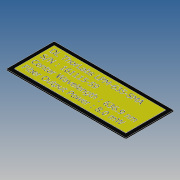
# Autodesk Inventor part: P131
Saved by Autodesk Inventor 2019 (Build 230136000, 136)
## iProperties
Created: 2017-01-31
Part Number: P131
Material: Generic
Document SubType Name: Modeling
Designer: serge.amoos
Density: 1 g/cm^3
Appearance: Smooth - Black
Description: Plaquette Thorlabs
Author: serge.amoos
Autodesk Inventor part; units mm, degrees
(part 1 of 3)
ref_plane "YZ Plane" through (0, 0, 0) normal (1, 0, 0) x (0, 1, 0)
ref_plane "XZ Plane" through (0, 0, 0) normal (0, 1, 0) x (-1, 0, 0)
ref_plane "XY Plane" through (0, 0, 0) normal (0, 0, 1) x (1, 0, 0)
sketch "Sketch1" plane through (0, 0, 0) normal (0, 0, 1) x (1, 0, 0)
  line L0 (-24.1301, 0) -> (24.0032, 0)
  line L1 (0, -8.4) -> (0, 8.4)
  line L2 (-15, 6) -> (15, 6)
  line L3 (15, 6) -> (15, -6)
  line L4 (15, -6) -> (-15, -6)
  line L5 (-15, -6) -> (-15, 6)
  point P0 (0, 0)
  point P1 (0, 6)
  point P2 (15, 0)
  dimension "d0" = 30
  dimension "d1" = 12
  constraints: 8 end point, 2 midpoint, 2 parallel, 2 point on line, 1 horizontal, 1 perpendicular
  measures "d0" distance of L2.start L2.end
  measures "d1" distance of L2.end L3.end
extrude "Extrusion1" add sketch "Sketch1" along normal blind 0.4
sketch "Sketch2" plane through (0, 0, 0.4) normal (0, 0, 1) x (1, 0, 0)
  line L0 (14, 5) -> (14, -5)
  line L1 (14, -5) -> (-14, -5)
  line L2 (-14, -5) -> (-14, 5)
  line L3 (-14, 5) -> (14, 5)
  line L4 (15, -6) -> (-15, -6)
  line L5 (-15, -6) -> (-15, 6)
  line L6 (-15, 6) -> (15, 6)
  line L7 (15, 6) -> (15, -6)
  point P0 (0, 0)
  dimension "d10" = 1
  dimension "d11" = 1
  dimension "d12" = 1
  dimension "d13" = 1
  constraints: 8 end point
  measures "d10" distance between parallel lines of L3 L6
  measures "d11" distance between parallel lines of L7 L0
  measures "d12" distance between parallel lines of L4 L1
  measures "d13" distance between parallel lines of L5 L2
extrude "Extrusion4" cut sketch "Sketch2" against normal blind 0.1
sketch "Sketch3" plane through (0, 0, 0.4) normal (0, 0, 1) x (1, 0, 0)
  line L0 (-13.4008, 7.7124) -> (17.127, 7.7124) construction
  line L1 (17.127, 7.7124) -> (17.127, -7.7124) construction
  line L2 (17.127, -7.7124) -> (-13.4008, -7.7124) construction
  line L3 (-13.4008, -7.7124) -> (-13.4008, 7.7124) construction
  line L4 (-23.9778, 0) -> (23.9778, 0)
  line L5 (0, -8.4) -> (0, 8.4)
  line L6 (14, -5) -> (-14, -5)
  line L7 (-14, -5) -> (-14, 5)
  line L8 (-14, 5) -> (14, 5)
  line L9 (14, 5) -> (14, -5)
  spline S0 degree 2 poles (-12.1551, 3.6187) (-12.1551, 3.427) (-12.3105, 3.1184) (-12.441, 3.0321) knots 0 0 0 1 2 2 2
  spline S1 degree 2 poles (-12.441, 3.0321) (-12.5477, 2.9652) (-12.7666, 2.9198) (-12.9368, 2.9198) knots 0 0 0 1 2 2 2
  line L10 (-12.9368, 2.9198) -> (-13.259, 2.9198)
  line L11 (-13.259, 2.9198) -> (-13.259, 4.3198)
  line L12 (-13.259, 4.3198) -> (-12.9402, 4.3198)
  spline S2 degree 2 poles (-12.9402, 4.3198) (-12.7428, 4.3198) (-12.5182, 4.2608) (-12.4387, 4.2086) knots 0 0 0 1 2 2 2
  spline S3 degree 2 poles (-12.4387, 4.2086) (-12.3037, 4.119) (-12.1551, 3.8229) (-12.1551, 3.6187) knots 0 0 0 1 2 2 2
  spline S4 degree 2 poles (-12.3491, 3.621) (-12.3491, 3.7821) (-12.4558, 4.0101) (-12.5613, 4.0748) knots 0 0 0 1 2 2 2
  spline S5 degree 2 poles (-12.5613, 4.0748) (-12.6362, 4.119) (-12.8052, 4.1587) (-12.9311, 4.1587) knots 0 0 0 1 2 2 2
  line L13 (-12.9311, 4.1587) -> (-13.0729, 4.1587)
  line L14 (-13.0729, 4.1587) -> (-13.0729, 3.0809)
  line L15 (-13.0729, 3.0809) -> (-12.9311, 3.0809)
  spline S6 degree 2 poles (-12.9311, 3.0809) (-12.8075, 3.0809) (-12.6203, 3.1206) (-12.5443, 3.174) knots 0 0 0 1 2 2 2
  spline S7 degree 2 poles (-12.5443, 3.174) (-12.4467, 3.2398) (-12.3491, 3.4576) (-12.3491, 3.621) knots 0 0 0 1 2 2 2
  line L16 (-11.142, 2.9198) -> (-11.9532, 2.9198)
  line L17 (-11.9532, 2.9198) -> (-11.9532, 4.3198)
  line L18 (-11.9532, 4.3198) -> (-11.7671, 4.3198)
  line L19 (-11.7671, 4.3198) -> (-11.7671, 3.0855)
  line L20 (-11.7671, 3.0855) -> (-11.142, 3.0855)
  line L21 (-11.142, 3.0855) -> (-11.142, 2.9198)
  line L22 (-10.0676, 2.9198) -> (-10.0676, 4.1542)
  line L23 (-10.0676, 4.1542) -> (-10.5373, 4.1542)
  line L24 (-10.5373, 4.1542) -> (-10.5373, 4.3198)
  line L25 (-10.5373, 4.3198) -> (-9.4118, 4.3198)
  line L26 (-9.4118, 4.3198) -> (-9.4118, 4.1542)
  line L27 (-9.4118, 4.1542) -> (-9.8815, 4.1542)
  line L28 (-9.8815, 4.1542) -> (-9.8815, 2.9198)
  line L29 (-9.8815, 2.9198) -> (-10.0676, 2.9198)
  line L30 (-8.4588, 2.9198) -> (-8.6358, 2.9198)
  line L31 (-8.6358, 2.9198) -> (-8.6358, 3.5189)
  spline S8 degree 2 poles (-8.6358, 3.5189) (-8.6358, 3.5915) (-8.6494, 3.7163) (-8.6699, 3.7537) knots 0 0 0 1 2 2 2
  spline S9 degree 2 poles (-8.6699, 3.7537) (-8.6914, 3.7934) (-8.7686, 3.832) (-8.8344, 3.832) knots 0 0 0 1 2 2 2
  spline S10 degree 2 poles (-8.8344, 3.832) (-8.9002, 3.832) (-9.0397, 3.7616) (-9.1067, 3.7049) knots 0 0 0 1 2 2 2
  line L32 (-9.1067, 3.7049) -> (-9.1067, 2.9198)
  line L33 (-9.1067, 2.9198) -> (-9.2836, 2.9198)
  line L34 (-9.2836, 2.9198) -> (-9.2836, 4.3822)
  line L35 (-9.2836, 4.3822) -> (-9.1067, 4.3822)
  line L36 (-9.1067, 4.3822) -> (-9.1067, 3.8535)
  spline S11 degree 2 poles (-9.1067, 3.8535) (-9.0272, 3.925) (-8.8741, 3.9999) (-8.7879, 3.9999) knots 0 0 0 1 2 2 2
  spline S12 degree 2 poles (-8.7879, 3.9999) (-8.6336, 3.9999) (-8.4588, 3.7957) (-8.4588, 3.6017) knots 0 0 0 1 2 2 2
  line L37 (-8.4588, 3.6017) -> (-8.4588, 2.9198)
  spline S13 degree 2 poles (-7.347, 3.4451) (-7.347, 3.1796) (-7.6023, 2.8903) (-7.8156, 2.8903) knots 0 0 0 1 2 2 2
  spline S14 degree 2 poles (-7.8156, 2.8903) (-8.0345, 2.8903) (-8.2853, 3.1887) (-8.2853, 3.4451) knots 0 0 0 1 2 2 2
  spline S15 degree 2 poles (-8.2853, 3.4451) (-8.2853, 3.7083) (-8.0266, 3.9999) (-7.8156, 3.9999) knots 0 0 0 1 2 2 2
  spline S16 degree 2 poles (-7.8156, 3.9999) (-7.6023, 3.9999) (-7.347, 3.7095) (-7.347, 3.4451) knots 0 0 0 1 2 2 2
  spline S17 degree 2 poles (-7.5297, 3.4451) (-7.5297, 3.6493) (-7.6783, 3.8479) (-7.8156, 3.8479) knots 0 0 0 1 2 2 2
  spline S18 degree 2 poles (-7.8156, 3.8479) (-7.9529, 3.8479) (-8.1026, 3.6493) (-8.1026, 3.4451) knots 0 0 0 1 2 2 2
  spline S19 degree 2 poles (-8.1026, 3.4451) (-8.1026, 3.2466) (-7.9529, 3.0424) (-7.8156, 3.0424) knots 0 0 0 1 2 2 2
  spline S20 degree 2 poles (-7.8156, 3.0424) (-7.6794, 3.0424) (-7.5297, 3.2432) (-7.5297, 3.4451) knots 0 0 0 1 2 2 2
  line L38 (-6.6084, 3.7809) -> (-6.6175, 3.7809)
  spline S21 degree 2 poles (-6.6175, 3.7809) (-6.6379, 3.7866) (-6.6822, 3.7889) (-6.7128, 3.7889) knots 0 0 0 1 2 2 2
  spline S22 degree 2 poles (-6.7128, 3.7889) (-6.7843, 3.7889) (-6.925, 3.7265) (-6.9885, 3.6652) knots 0 0 0 1 2 2 2
  line L39 (-6.9885, 3.6652) -> (-6.9885, 2.9198)
  line L40 (-6.9885, 2.9198) -> (-7.1655, 2.9198)
  line L41 (-7.1655, 2.9198) -> (-7.1655, 3.9704)
  line L42 (-7.1655, 3.9704) -> (-6.9885, 3.9704)
  line L43 (-6.9885, 3.9704) -> (-6.9885, 3.8138)
  spline S23 degree 2 poles (-6.9885, 3.8138) (-6.8921, 3.9001) (-6.748, 3.9704) (-6.6799, 3.9704) knots 0 0 0 1 2 2 2
  spline S24 degree 2 poles (-6.6799, 3.9704) (-6.6527, 3.9704) (-6.6255, 3.9681) (-6.6084, 3.9647) knots 0 0 0 1 2 2 2
  line L44 (-6.6084, 3.9647) -> (-6.6084, 3.7809)
  line L45 (-5.6464, 2.9198) -> (-6.4576, 2.9198)
  line L46 (-6.4576, 2.9198) -> (-6.4576, 4.3198)
  line L47 (-6.4576, 4.3198) -> (-6.2715, 4.3198)
  line L48 (-6.2715, 4.3198) -> (-6.2715, 3.0855)
  line L49 (-6.2715, 3.0855) -> (-5.6464, 3.0855)
  line L50 (-5.6464, 3.0855) -> (-5.6464, 2.9198)
  spline S25 degree 2 poles (-4.9282, 3.031) (-4.9498, 3.0151) (-5.0224, 2.9584) (-5.0564, 2.9414) knots 0 0 0 1 2 2 2
  spline S26 degree 2 poles (-5.0564, 2.9414) (-5.1029, 2.9164) (-5.1903, 2.8903) (-5.2697, 2.8903) knots 0 0 0 1 2 2 2
  spline S27 degree 2 poles (-5.2697, 2.8903) (-5.3344, 2.8903) (-5.4512, 2.9391) (-5.4955, 2.9834) knots 0 0 0 1 2 2 2
  spline S28 degree 2 poles (-5.4955, 2.9834) (-5.5375, 3.0265) (-5.5885, 3.1535) (-5.5885, 3.2239) knots 0 0 0 1 2 2 2
  spline S29 degree 2 poles (-5.5885, 3.2239) (-5.5885, 3.3328) (-5.4966, 3.4871) (-5.3968, 3.5313) knots 0 0 0 1 2 2 2
  spline S30 degree 2 poles (-5.3968, 3.5313) (-5.3083, 3.5722) (-5.0678, 3.6028) (-4.9282, 3.6108) knots 0 0 0 1 2 2 2
  line L51 (-4.9282, 3.6108) -> (-4.9282, 3.6448)
  spline S31 degree 2 poles (-4.9282, 3.6448) (-4.9282, 3.7061) (-4.9657, 3.7821) (-4.9997, 3.8036) knots 0 0 0 1 2 2 2
  spline S32 degree 2 poles (-4.9997, 3.8036) (-5.0337, 3.8252) (-5.1313, 3.8388) (-5.1835, 3.8388) knots 0 0 0 1 2 2 2
  spline S33 degree 2 poles (-5.1835, 3.8388) (-5.2447, 3.8388) (-5.4104, 3.8025) (-5.4932, 3.7673) knots 0 0 0 1 2 2 2
  line L52 (-5.4932, 3.7673) -> (-5.5034, 3.7673)
  line L53 (-5.5034, 3.7673) -> (-5.5034, 3.9477)
  spline S34 degree 2 poles (-5.5034, 3.9477) (-5.4546, 3.9613) (-5.272, 3.9954) (-5.1823, 3.9954) knots 0 0 0 1 2 2 2
  spline S35 degree 2 poles (-5.1823, 3.9954) (-5.0734, 3.9954) (-4.9248, 3.9613) (-4.8658, 3.9171) knots 0 0 0 1 2 2 2
  spline S36 degree 2 poles (-4.8658, 3.9171) (-4.808, 3.874) (-4.7512, 3.7367) (-4.7512, 3.638) knots 0 0 0 1 2 2 2
  line L54 (-4.7512, 3.638) -> (-4.7512, 2.9198)
  line L55 (-4.7512, 2.9198) -> (-4.9282, 2.9198)
  line L56 (-4.9282, 2.9198) -> (-4.9282, 3.031)
  line L57 (-4.9282, 3.1785) -> (-4.9282, 3.4701)
  spline S37 degree 2 poles (-4.9282, 3.4701) (-4.9917, 3.4644) (-5.1835, 3.4451) (-5.2436, 3.427) knots 0 0 0 1 2 2 2
  spline S38 degree 2 poles (-5.2436, 3.427) (-5.314, 3.4054) (-5.4058, 3.3158) (-5.4058, 3.2364) knots 0 0 0 1 2 2 2
  spline S39 degree 2 poles (-5.4058, 3.2364) (-5.4058, 3.1456) (-5.3037, 3.0537) (-5.2062, 3.0537) knots 0 0 0 1 2 2 2
  spline S40 degree 2 poles (-5.2062, 3.0537) (-5.1234, 3.0537) (-4.9872, 3.1252) (-4.9282, 3.1785) knots 0 0 0 1 2 2 2
  spline S41 degree 2 poles (-3.6224, 3.4621) (-3.6224, 3.2046) (-3.872, 2.8903) (-4.0603, 2.8903) knots 0 0 0 1 2 2 2
  spline S42 degree 2 poles (-4.0603, 2.8903) (-4.1454, 2.8903) (-4.2668, 2.9323) (-4.3258, 2.9686) knots 0 0 0 1 2 2 2
  line L58 (-4.3258, 2.9686) -> (-4.3371, 2.9198)
  line L59 (-4.3371, 2.9198) -> (-4.5028, 2.9198)
  line L60 (-4.5028, 2.9198) -> (-4.5028, 4.3822)
  line L61 (-4.5028, 4.3822) -> (-4.3258, 4.3822)
  line L62 (-4.3258, 4.3822) -> (-4.3258, 3.8603)
  spline S43 degree 2 poles (-4.3258, 3.8603) (-4.2588, 3.9205) (-4.1034, 3.9999) (-4.0047, 3.9999) knots 0 0 0 1 2 2 2
  spline S44 degree 2 poles (-4.0047, 3.9999) (-3.8266, 3.9999) (-3.6224, 3.7151) (-3.6224, 3.4621) knots 0 0 0 1 2 2 2
  spline S45 degree 2 poles (-3.805, 3.4485) (-3.805, 3.6368) (-3.9196, 3.832) (-4.0467, 3.832) knots 0 0 0 1 2 2 2
  spline S46 degree 2 poles (-4.0467, 3.832) (-4.1182, 3.832) (-4.2657, 3.7639) (-4.3258, 3.7117) knots 0 0 0 1 2 2 2
  line L63 (-4.3258, 3.7117) -> (-4.3258, 3.1093)
  spline S47 degree 2 poles (-4.3258, 3.1093) (-4.2588, 3.0764) (-4.1556, 3.0492) (-4.0943, 3.0492) knots 0 0 0 1 2 2 2
  spline S48 degree 2 poles (-4.0943, 3.0492) (-3.9593, 3.0492) (-3.805, 3.2409) (-3.805, 3.4485) knots 0 0 0 1 2 2 2
  spline S49 degree 2 poles (-3.155, 2.8949) (-3.2605, 2.8949) (-3.4431, 2.9516) (-3.5033, 2.9834) knots 0 0 0 1 2 2 2
  line L64 (-3.5033, 2.9834) -> (-3.5033, 3.1819)
  line L65 (-3.5033, 3.1819) -> (-3.4942, 3.1819)
  spline S50 degree 2 poles (-3.4942, 3.1819) (-3.4715, 3.1638) (-3.4102, 3.1206) (-3.3592, 3.0968) knots 0 0 0 1 2 2 2
  spline S51 degree 2 poles (-3.3592, 3.0968) (-3.3149, 3.0753) (-3.206, 3.0435) (-3.1482, 3.0435) knots 0 0 0 1 2 2 2
  spline S52 degree 2 poles (-3.1482, 3.0435) (-3.1062, 3.0435) (-3.0097, 3.0628) (-2.987, 3.0787) knots 0 0 0 1 2 2 2
  spline S53 degree 2 poles (-2.987, 3.0787) (-2.9541, 3.1002) (-2.9246, 3.149) (-2.9246, 3.1989) knots 0 0 0 1 2 2 2
  spline S54 degree 2 poles (-2.9246, 3.1989) (-2.9246, 3.2613) (-2.9927, 3.326) (-3.0801, 3.3475) knots 0 0 0 1 2 2 2
  spline S55 degree 2 poles (-3.0801, 3.3475) (-3.1141, 3.3555) (-3.223, 3.3782) (-3.2695, 3.3907) knots 0 0 0 1 2 2 2
  spline S56 degree 2 poles (-3.2695, 3.3907) (-3.3898, 3.4258) (-3.4987, 3.571) (-3.4987, 3.6743) knots 0 0 0 1 2 2 2
  spline S57 degree 2 poles (-3.4987, 3.6743) (-3.4987, 3.8172) (-3.2843, 3.9954) (-3.1073, 3.9954) knots 0 0 0 1 2 2 2
  spline S58 degree 2 poles (-3.1073, 3.9954) (-3.0199, 3.9954) (-2.843, 3.9522) (-2.7828, 3.9193) knots 0 0 0 1 2 2 2
  line L66 (-2.7828, 3.9193) -> (-2.7828, 3.7299)
  line L67 (-2.7828, 3.7299) -> (-2.7919, 3.7299)
  spline S59 degree 2 poles (-2.7919, 3.7299) (-2.86, 3.7843) (-3.0256, 3.8467) (-3.1107, 3.8467) knots 0 0 0 1 2 2 2
  spline S60 degree 2 poles (-3.1107, 3.8467) (-3.1981, 3.8467) (-3.3183, 3.773) (-3.3183, 3.6992) knots 0 0 0 1 2 2 2
  spline S61 degree 2 poles (-3.3183, 3.6992) (-3.3183, 3.6323) (-3.2469, 3.5676) (-3.1674, 3.5472) knots 0 0 0 1 2 2 2
  spline S62 degree 2 poles (-3.1674, 3.5472) (-3.1289, 3.537) (-3.0313, 3.5166) (-2.978, 3.5041) knots 0 0 0 1 2 2 2
  spline S63 degree 2 poles (-2.978, 3.5041) (-2.8623, 3.4746) (-2.7443, 3.3396) (-2.7443, 3.2227) knots 0 0 0 1 2 2 2
  spline S64 degree 2 poles (-2.7443, 3.2227) (-2.7443, 3.1547) (-2.7976, 3.0344) (-2.8498, 2.9902) knots 0 0 0 1 2 2 2
  spline S65 degree 2 poles (-2.8498, 2.9902) (-2.9054, 2.9437) (-3.0472, 2.8949) (-3.155, 2.8949) knots 0 0 0 1 2 2 2
  line L68 (-1.1537, 2.9198) -> (-1.9648, 2.9198)
  line L69 (-1.9648, 2.9198) -> (-1.9648, 4.3198)
  line L70 (-1.9648, 4.3198) -> (-1.7788, 4.3198)
  line L71 (-1.7788, 4.3198) -> (-1.7788, 3.0855)
  line L72 (-1.7788, 3.0855) -> (-1.1537, 3.0855)
  line L73 (-1.1537, 3.0855) -> (-1.1537, 2.9198)
  spline S66 degree 2 poles (-0.1224, 3.8978) (-0.1224, 3.807) (-0.187, 3.6437) (-0.2449, 3.5869) knots 0 0 0 1 2 2 2
  spline S67 degree 2 poles (-0.2449, 3.5869) (-0.3175, 3.5155) (-0.5138, 3.4417) (-0.6635, 3.4417) knots 0 0 0 1 2 2 2
  line L74 (-0.6635, 3.4417) -> (-0.8212, 3.4417)
  line L75 (-0.8212, 3.4417) -> (-0.8212, 2.9198)
  line L76 (-0.8212, 2.9198) -> (-1.0073, 2.9198)
  line L77 (-1.0073, 2.9198) -> (-1.0073, 4.3198)
  line L78 (-1.0073, 4.3198) -> (-0.6556, 4.3198)
  spline S68 degree 2 poles (-0.6556, 4.3198) (-0.5308, 4.3198) (-0.3561, 4.279) (-0.2892, 4.2325) knots 0 0 0 1 2 2 2
  spline S69 degree 2 poles (-0.2892, 4.2325) (-0.2109, 4.1792) (-0.1224, 4.0146) (-0.1224, 3.8978) knots 0 0 0 1 2 2 2
  spline S70 degree 2 poles (-0.3164, 3.8921) (-0.3164, 3.9647) (-0.3663, 4.0714) (-0.4174, 4.1054) knots 0 0 0 1 2 2 2
  spline S71 degree 2 poles (-0.4174, 4.1054) (-0.4616, 4.1349) (-0.5796, 4.1587) (-0.667, 4.1587) knots 0 0 0 1 2 2 2
  line L79 (-0.667, 4.1587) -> (-0.8212, 4.1587)
  line L80 (-0.8212, 4.1587) -> (-0.8212, 3.6005)
  line L81 (-0.8212, 3.6005) -> (-0.6942, 3.6005)
  spline S72 degree 2 poles (-0.6942, 3.6005) (-0.5807, 3.6005) (-0.4412, 3.6368) (-0.3958, 3.6845) knots 0 0 0 1 2 2 2
  spline S73 degree 2 poles (-0.3958, 3.6845) (-0.3538, 3.7265) (-0.3164, 3.8252) (-0.3164, 3.8921) knots 0 0 0 1 2 2 2
  line L82 (1.2549, 2.9198) -> (1.0689, 2.9198)
  line L83 (1.0689, 2.9198) -> (1.0689, 4.1258)
  line L84 (1.0689, 4.1258) -> (0.7036, 3.3056)
  line L85 (0.7036, 3.3056) -> (0.5901, 3.3056)
  line L86 (0.5901, 3.3056) -> (0.2282, 4.1258)
  line L87 (0.2282, 4.1258) -> (0.2282, 2.9198)
  line L88 (0.2282, 2.9198) -> (0.0546, 2.9198)
  line L89 (0.0546, 2.9198) -> (0.0546, 4.3198)
  line L90 (0.0546, 4.3198) -> (0.3087, 4.3198)
  line L91 (0.3087, 4.3198) -> (0.6582, 3.5404)
  line L92 (0.6582, 3.5404) -> (0.9963, 4.3198)
  line L93 (0.9963, 4.3198) -> (1.2549, 4.3198)
  line L94 (1.2549, 4.3198) -> (1.2549, 2.9198)
  line L95 (2.0117, 3.4474) -> (1.4818, 3.4474)
  line L96 (1.4818, 3.4474) -> (1.4818, 3.6176)
  line L97 (1.4818, 3.6176) -> (2.0117, 3.6176)
  line L98 (2.0117, 3.6176) -> (2.0117, 3.4474)
  spline S74 degree 2 poles (3.0826, 3.3736) (3.0826, 3.2659) (3.0112, 3.0832) (2.951, 3.0219) knots 0 0 0 1 2 2 2
  spline S75 degree 2 poles (2.951, 3.0219) (2.8886, 2.9573) (2.7321, 2.8903) (2.6379, 2.8903) knots 0 0 0 1 2 2 2
  spline S76 degree 2 poles (2.6379, 2.8903) (2.5437, 2.8903) (2.3883, 2.9539) (2.3293, 3.0174) knots 0 0 0 1 2 2 2
  spline S77 degree 2 poles (2.3293, 3.0174) (2.2567, 3.0934) (2.175, 3.3487) (2.175, 3.5347) knots 0 0 0 1 2 2 2
  spline S78 degree 2 poles (2.175, 3.5347) (2.175, 3.7174) (2.2499, 4.0112) (2.3282, 4.1202) knots 0 0 0 1 2 2 2
  spline S79 degree 2 poles (2.3282, 4.1202) (2.4042, 4.2268) (2.6447, 4.3459) (2.8024, 4.3459) knots 0 0 0 1 2 2 2
  spline S80 degree 2 poles (2.8024, 4.3459) (2.8489, 4.3459) (2.9306, 4.3368) (2.9613, 4.3266) knots 0 0 0 1 2 2 2
  line L99 (2.9613, 4.3266) -> (2.9613, 4.1462)
  line L100 (2.9613, 4.1462) -> (2.9533, 4.1462)
  spline S81 degree 2 poles (2.9533, 4.1462) (2.9272, 4.1599) (2.8319, 4.1837) (2.7775, 4.1837) knots 0 0 0 1 2 2 2
  spline S82 degree 2 poles (2.7775, 4.1837) (2.6027, 4.1837) (2.3883, 3.9477) (2.3679, 3.7163) knots 0 0 0 1 2 2 2
  spline S83 degree 2 poles (2.3679, 3.7163) (2.4348, 3.7628) (2.5755, 3.8138) (2.6595, 3.8138) knots 0 0 0 1 2 2 2
  spline S84 degree 2 poles (2.6595, 3.8138) (2.7412, 3.8138) (2.8637, 3.7809) (2.9306, 3.731) knots 0 0 0 1 2 2 2
  spline S85 degree 2 poles (2.9306, 3.731) (3.0078, 3.6732) (3.0826, 3.4939) (3.0826, 3.3736) knots 0 0 0 1 2 2 2
  spline S86 degree 2 poles (2.892, 3.3657) (2.892, 3.4519) (2.8467, 3.5688) (2.7967, 3.6096) knots 0 0 0 1 2 2 2
  spline S87 degree 2 poles (2.7967, 3.6096) (2.7593, 3.6391) (2.6663, 3.6584) (2.6175, 3.6584) knots 0 0 0 1 2 2 2
  spline S88 degree 2 poles (2.6175, 3.6584) (2.5517, 3.6584) (2.428, 3.6187) (2.3679, 3.5813) knots 0 0 0 1 2 2 2
  spline S89 degree 2 poles (2.3679, 3.5813) (2.3668, 3.5608) (2.3645, 3.5223) (2.3645, 3.4928) knots 0 0 0 1 2 2 2
  spline S90 degree 2 poles (2.3645, 3.4928) (2.3645, 3.3475) (2.4212, 3.1694) (2.4643, 3.1229) knots 0 0 0 1 2 2 2
  spline S91 degree 2 poles (2.4643, 3.1229) (2.504, 3.0787) (2.5903, 3.0435) (2.639, 3.0435) knots 0 0 0 1 2 2 2
  spline S92 degree 2 poles (2.639, 3.0435) (2.7525, 3.0435) (2.892, 3.2046) (2.892, 3.3657) knots 0 0 0 1 2 2 2
  spline S93 degree 2 poles (3.6261, 4.1871) (3.575, 4.1871) (3.4741, 4.1621) (3.4253, 4.1428) knots 0 0 0 1 2 2 2
  spline S94 degree 2 poles (3.4253, 4.1428) (3.3799, 4.1236) (3.313, 4.0827) (3.2869, 4.0646) knots 0 0 0 1 2 2 2
  line L101 (3.2869, 4.0646) -> (3.2755, 4.0646)
  line L102 (3.2755, 4.0646) -> (3.2755, 4.2631)
  spline S95 degree 2 poles (3.2755, 4.2631) (3.3368, 4.296) (3.5467, 4.3493) (3.6408, 4.3493) knots 0 0 0 1 2 2 2
  spline S96 degree 2 poles (3.6408, 4.3493) (3.7361, 4.3493) (3.8779, 4.3108) (3.9358, 4.2699) knots 0 0 0 1 2 2 2
  spline S97 degree 2 poles (3.9358, 4.2699) (3.9971, 4.2257) (4.0606, 4.0975) (4.0606, 4.0112) knots 0 0 0 1 2 2 2
  spline S98 degree 2 poles (4.0606, 4.0112) (4.0606, 3.8955) (3.9086, 3.7208) (3.8019, 3.6981) knots 0 0 0 1 2 2 2
  line L103 (3.8019, 3.6981) -> (3.8019, 3.6845)
  spline S99 degree 2 poles (3.8019, 3.6845) (3.8462, 3.6754) (3.9471, 3.6346) (3.9903, 3.5937) knots 0 0 0 1 2 2 2
  spline S100 degree 2 poles (3.9903, 3.5937) (4.0334, 3.554) (4.0878, 3.427) (4.0878, 3.3351) knots 0 0 0 1 2 2 2
  spline S101 degree 2 poles (4.0878, 3.3351) (4.0878, 3.2409) (4.0232, 3.0809) (3.9642, 3.0197) knots 0 0 0 1 2 2 2
  spline S102 degree 2 poles (3.9642, 3.0197) (3.9029, 2.9561) (3.7293, 2.8903) (3.6193, 2.8903) knots 0 0 0 1 2 2 2
  spline S103 degree 2 poles (3.6193, 2.8903) (3.5138, 2.8903) (3.3073, 2.9414) (3.2369, 2.9766) knots 0 0 0 1 2 2 2
  line L104 (3.2369, 2.9766) -> (3.2369, 3.1751)
  line L105 (3.2369, 3.1751) -> (3.2506, 3.1751)
  spline S104 degree 2 poles (3.2506, 3.1751) (3.3095, 3.132) (3.5092, 3.0526) (3.6079, 3.0526) knots 0 0 0 1 2 2 2
  spline S105 degree 2 poles (3.6079, 3.0526) (3.6658, 3.0526) (3.7815, 3.0889) (3.8201, 3.1309) knots 0 0 0 1 2 2 2
  spline S106 degree 2 poles (3.8201, 3.1309) (3.8575, 3.1728) (3.8972, 3.2727) (3.8972, 3.3487) knots 0 0 0 1 2 2 2
  spline S107 degree 2 poles (3.8972, 3.3487) (3.8972, 3.4247) (3.853, 3.5234) (3.8133, 3.5518) knots 0 0 0 1 2 2 2
  spline S108 degree 2 poles (3.8133, 3.5518) (3.7736, 3.5801) (3.6658, 3.6017) (3.6023, 3.6017) knots 0 0 0 1 2 2 2
  line L106 (3.6023, 3.6017) -> (3.5228, 3.6017)
  line L107 (3.5228, 3.6017) -> (3.5228, 3.7571)
  line L108 (3.5228, 3.7571) -> (3.5852, 3.7571)
  spline S109 degree 2 poles (3.5852, 3.7571) (3.7112, 3.7571) (3.87, 3.8774) (3.87, 3.992) knots 0 0 0 1 2 2 2
  spline S110 degree 2 poles (3.87, 3.992) (3.87, 4.0453) (3.8292, 4.1213) (3.7963, 4.144) knots 0 0 0 1 2 2 2
  spline S111 degree 2 poles (3.7963, 4.144) (3.7611, 4.1678) (3.6749, 4.1871) (3.6261, 4.1871) knots 0 0 0 1 2 2 2
  spline S112 degree 2 poles (5.1475, 3.3646) (5.1475, 3.2636) (5.0828, 3.0911) (5.0238, 3.0276) knots 0 0 0 1 2 2 2
  spline S113 degree 2 poles (5.0238, 3.0276) (4.9648, 2.9641) (4.789, 2.8903) (4.6801, 2.8903) knots 0 0 0 1 2 2 2
  spline S114 degree 2 poles (4.6801, 2.8903) (4.5802, 2.8903) (4.3851, 2.9346) (4.3136, 2.9698) knots 0 0 0 1 2 2 2
  line L109 (4.3136, 2.9698) -> (4.3136, 3.1683)
  line L110 (4.3136, 3.1683) -> (4.3272, 3.1683)
  spline S115 degree 2 poles (4.3272, 3.1683) (4.3488, 3.1524) (4.4293, 3.1116) (4.4781, 3.0934) knots 0 0 0 1 2 2 2
  spline S116 degree 2 poles (4.4781, 3.0934) (4.5337, 3.0741) (4.6256, 3.0526) (4.6835, 3.0526) knots 0 0 0 1 2 2 2
  spline S117 degree 2 poles (4.6835, 3.0526) (4.7402, 3.0526) (4.8468, 3.0934) (4.8854, 3.1377) knots 0 0 0 1 2 2 2
  spline S118 degree 2 poles (4.8854, 3.1377) (4.9206, 3.1796) (4.9569, 3.2908) (4.9569, 3.3657) knots 0 0 0 1 2 2 2
  spline S119 degree 2 poles (4.9569, 3.3657) (4.9569, 3.4406) (4.916, 3.5359) (4.8775, 3.5676) knots 0 0 0 1 2 2 2
  spline S120 degree 2 poles (4.8775, 3.5676) (4.8377, 3.6028) (4.7198, 3.6323) (4.6483, 3.6323) knots 0 0 0 1 2 2 2
  spline S121 degree 2 poles (4.6483, 3.6323) (4.5711, 3.6323) (4.418, 3.6085) (4.3715, 3.5983) knots 0 0 0 1 2 2 2
  line L111 (4.3715, 3.5983) -> (4.3715, 4.3198)
  line L112 (4.3715, 4.3198) -> (5.1395, 4.3198)
  line L113 (5.1395, 4.3198) -> (5.1395, 4.1553)
  line L114 (5.1395, 4.1553) -> (4.5518, 4.1553)
  line L115 (4.5518, 4.1553) -> (4.5518, 3.7821)
  spline S122 degree 2 poles (4.5518, 3.7821) (4.5859, 3.7866) (4.6517, 3.79) (4.6789, 3.79) knots 0 0 0 1 2 2 2
  spline S123 degree 2 poles (4.6789, 3.79) (4.7867, 3.79) (4.9353, 3.7548) (5.0034, 3.7027) knots 0 0 0 1 2 2 2
  spline S124 degree 2 poles (5.0034, 3.7027) (5.0726, 3.6505) (5.1475, 3.4916) (5.1475, 3.3646) knots 0 0 0 1 2 2 2
  line L116 (5.8622, 3.4474) -> (5.3324, 3.4474)
  line L117 (5.3324, 3.4474) -> (5.3324, 3.6176)
  line L118 (5.3324, 3.6176) -> (5.8622, 3.6176)
  line L119 (5.8622, 3.6176) -> (5.8622, 3.4474)
  spline S125 degree 2 poles (6.4783, 2.8949) (6.3262, 2.8949) (6.113, 2.9584) (6.0188, 3.0038) knots 0 0 0 1 2 2 2
  line L120 (6.0188, 3.0038) -> (6.0188, 3.2375)
  line L121 (6.0188, 3.2375) -> (6.0324, 3.2375)
  spline S126 degree 2 poles (6.0324, 3.2375) (6.1243, 3.1513) (6.3569, 3.056) (6.4647, 3.056) knots 0 0 0 1 2 2 2
  spline S127 degree 2 poles (6.4647, 3.056) (6.6189, 3.056) (6.7766, 3.1842) (6.7766, 3.2897) knots 0 0 0 1 2 2 2
  spline S128 degree 2 poles (6.7766, 3.2897) (6.7766, 3.3736) (6.6938, 3.478) (6.6042, 3.5041) knots 0 0 0 1 2 2 2
  spline S129 degree 2 poles (6.6042, 3.5041) (6.5395, 3.5223) (6.4318, 3.5472) (6.3512, 3.5676) knots 0 0 0 1 2 2 2
  spline S130 degree 2 poles (6.3512, 3.5676) (6.2786, 3.5869) (6.164, 3.6448) (6.1198, 3.6913) knots 0 0 0 1 2 2 2
  spline S131 degree 2 poles (6.1198, 3.6913) (6.0766, 3.7378) (6.029, 3.8626) (6.029, 3.9443) knots 0 0 0 1 2 2 2
  spline S132 degree 2 poles (6.029, 3.9443) (6.029, 4.1145) (6.2945, 4.3448) (6.4998, 4.3448) knots 0 0 0 1 2 2 2
  spline S133 degree 2 poles (6.4998, 4.3448) (6.6178, 4.3448) (6.8266, 4.2983) (6.9162, 4.254) knots 0 0 0 1 2 2 2
  line L122 (6.9162, 4.254) -> (6.9162, 4.0317)
  line L123 (6.9162, 4.0317) -> (6.9026, 4.0317)
  spline S134 degree 2 poles (6.9026, 4.0317) (6.8356, 4.0929) (6.6269, 4.1837) (6.5123, 4.1837) knots 0 0 0 1 2 2 2
  spline S135 degree 2 poles (6.5123, 4.1837) (6.383, 4.1837) (6.223, 4.0623) (6.223, 3.9636) knots 0 0 0 1 2 2 2
  spline S136 degree 2 poles (6.223, 3.9636) (6.223, 3.8751) (6.3172, 3.7696) (6.4057, 3.7458) knots 0 0 0 1 2 2 2
  spline S137 degree 2 poles (6.4057, 3.7458) (6.4647, 3.7299) (6.636, 3.689) (6.6927, 3.672) knots 0 0 0 1 2 2 2
  spline S138 degree 2 poles (6.6927, 3.672) (6.8368, 3.6278) (6.9707, 3.4497) (6.9707, 3.3192) knots 0 0 0 1 2 2 2
  spline S139 degree 2 poles (6.9707, 3.3192) (6.9707, 3.2364) (6.9037, 3.0775) (6.8436, 3.0219) knots 0 0 0 1 2 2 2
  spline S140 degree 2 poles (6.8436, 3.0219) (6.7766, 2.9607) (6.6065, 2.8949) (6.4783, 2.8949) knots 0 0 0 1 2 2 2
  line L124 (8.3604, 2.9198) -> (8.1744, 2.9198)
  line L125 (8.1744, 2.9198) -> (8.1744, 4.1258)
  line L126 (8.1744, 4.1258) -> (7.8091, 3.3056)
  line L127 (7.8091, 3.3056) -> (7.6956, 3.3056)
  line L128 (7.6956, 3.3056) -> (7.3337, 4.1258)
  line L129 (7.3337, 4.1258) -> (7.3337, 2.9198)
  line L130 (7.3337, 2.9198) -> (7.1601, 2.9198)
  line L131 (7.1601, 2.9198) -> (7.1601, 4.3198)
  line L132 (7.1601, 4.3198) -> (7.4142, 4.3198)
  line L133 (7.4142, 4.3198) -> (7.7637, 3.5404)
  line L134 (7.7637, 3.5404) -> (8.1018, 4.3198)
  line L135 (8.1018, 4.3198) -> (8.3604, 4.3198)
  line L136 (8.3604, 4.3198) -> (8.3604, 2.9198)
  line L137 (8.4932, 2.9198) -> (8.9651, 4.3198)
  line L138 (8.9651, 4.3198) -> (9.1943, 4.3198)
  line L139 (9.1943, 4.3198) -> (9.6663, 2.9198)
  line L140 (9.6663, 2.9198) -> (9.47, 2.9198)
  line L141 (9.47, 2.9198) -> (9.3429, 3.3112)
  line L142 (9.3429, 3.3112) -> (8.8086, 3.3112)
  line L143 (8.8086, 3.3112) -> (8.6815, 2.9198)
  line L144 (8.6815, 2.9198) -> (8.4932, 2.9198)
  line L145 (9.2919, 3.4701) -> (9.0752, 4.1292)
  line L146 (9.0752, 4.1292) -> (8.8596, 3.4701)
  line L147 (8.8596, 3.4701) -> (9.2919, 3.4701)
  spline S141 degree 2 poles (-12.8687, 0.5898) (-13.0208, 0.5898) (-13.234, 0.6533) (-13.3282, 0.6987) knots 0 0 0 1 2 2 2
  line L148 (-13.3282, 0.6987) -> (-13.3282, 0.9324)
  line L149 (-13.3282, 0.9324) -> (-13.3146, 0.9324)
  spline S142 degree 2 poles (-13.3146, 0.9324) (-13.2227, 0.8462) (-12.9901, 0.7509) (-12.8823, 0.7509) knots 0 0 0 1 2 2 2
  spline S143 degree 2 poles (-12.8823, 0.7509) (-12.7281, 0.7509) (-12.5704, 0.8791) (-12.5704, 0.9846) knots 0 0 0 1 2 2 2
  spline S144 degree 2 poles (-12.5704, 0.9846) (-12.5704, 1.0686) (-12.6532, 1.173) (-12.7428, 1.199) knots 0 0 0 1 2 2 2
  spline S145 degree 2 poles (-12.7428, 1.199) (-12.8075, 1.2172) (-12.9152, 1.2422) (-12.9958, 1.2626) knots 0 0 0 1 2 2 2
  spline S146 degree 2 poles (-12.9958, 1.2626) (-13.0684, 1.2819) (-13.183, 1.3397) (-13.2272, 1.3862) knots 0 0 0 1 2 2 2
  spline S147 degree 2 poles (-13.2272, 1.3862) (-13.2704, 1.4328) (-13.318, 1.5576) (-13.318, 1.6392) knots 0 0 0 1 2 2 2
  spline S148 degree 2 poles (-13.318, 1.6392) (-13.318, 1.8094) (-13.0525, 2.0397) (-12.8472, 2.0397) knots 0 0 0 1 2 2 2
  spline S149 degree 2 poles (-12.8472, 2.0397) (-12.7292, 2.0397) (-12.5204, 1.9932) (-12.4308, 1.949) knots 0 0 0 1 2 2 2
  line L150 (-12.4308, 1.949) -> (-12.4308, 1.7266)
  line L151 (-12.4308, 1.7266) -> (-12.4444, 1.7266)
  spline S150 degree 2 poles (-12.4444, 1.7266) (-12.5114, 1.7879) (-12.7201, 1.8786) (-12.8347, 1.8786) knots 0 0 0 1 2 2 2
  spline S151 degree 2 poles (-12.8347, 1.8786) (-12.964, 1.8786) (-13.124, 1.7572) (-13.124, 1.6585) knots 0 0 0 1 2 2 2
  spline S152 degree 2 poles (-13.124, 1.6585) (-13.124, 1.57) (-13.0298, 1.4645) (-12.9413, 1.4407) knots 0 0 0 1 2 2 2
  spline S153 degree 2 poles (-12.9413, 1.4407) (-12.8823, 1.4248) (-12.711, 1.384) (-12.6543, 1.367) knots 0 0 0 1 2 2 2
  spline S154 degree 2 poles (-12.6543, 1.367) (-12.5102, 1.3227) (-12.3764, 1.1446) (-12.3764, 1.0141) knots 0 0 0 1 2 2 2
  spline S155 degree 2 poles (-12.3764, 1.0141) (-12.3764, 0.9313) (-12.4433, 0.7725) (-12.5034, 0.7169) knots 0 0 0 1 2 2 2
  spline S156 degree 2 poles (-12.5034, 0.7169) (-12.5704, 0.6556) (-12.7405, 0.5898) (-12.8687, 0.5898) knots 0 0 0 1 2 2 2
  line L152 (-11.6446, 2.0772) -> (-12.1926, 0.3107)
  line L153 (-12.1926, 0.3107) -> (-12.3514, 0.3107)
  line L154 (-12.3514, 0.3107) -> (-11.8057, 2.0772)
  line L155 (-11.8057, 2.0772) -> (-11.6446, 2.0772)
  line L156 (-10.4488, 0.6148) -> (-10.6576, 0.6148)
  line L157 (-10.6576, 0.6148) -> (-11.277, 1.8219)
  line L158 (-11.277, 1.8219) -> (-11.277, 0.6148)
  line L159 (-11.277, 0.6148) -> (-11.4506, 0.6148)
  line L160 (-11.4506, 0.6148) -> (-11.4506, 2.0148)
  line L161 (-11.4506, 2.0148) -> (-11.1862, 2.0148)
  line L162 (-11.1862, 2.0148) -> (-10.6224, 0.9063)
  line L163 (-10.6224, 0.9063) -> (-10.6224, 2.0148)
  line L164 (-10.6224, 2.0148) -> (-10.4488, 2.0148)
  line L165 (-10.4488, 2.0148) -> (-10.4488, 0.6148)
  line L166 (-9.253, 1.3976) -> (-9.4776, 1.3976)
  line L167 (-9.4776, 1.3976) -> (-9.4776, 1.6653)
  line L168 (-9.4776, 1.6653) -> (-9.253, 1.6653)
  line L169 (-9.253, 1.6653) -> (-9.253, 1.3976)
  line L170 (-9.253, 0.6148) -> (-9.4776, 0.6148)
  line L171 (-9.4776, 0.6148) -> (-9.4776, 0.8825)
  line L172 (-9.4776, 0.8825) -> (-9.253, 0.8825)
  line L173 (-9.253, 0.8825) -> (-9.253, 0.6148)
  line L174 (-7.5285, 0.6148) -> (-8.2115, 0.6148)
  line L175 (-8.2115, 0.6148) -> (-8.2115, 0.7577)
  line L176 (-8.2115, 0.7577) -> (-7.9574, 0.7577)
  line L177 (-7.9574, 0.7577) -> (-7.9574, 1.696)
  line L178 (-7.9574, 1.696) -> (-8.2115, 1.696)
  line L179 (-8.2115, 1.696) -> (-8.2115, 1.8242)
  spline S157 degree 2 poles (-8.2115, 1.8242) (-8.0674, 1.8242) (-7.9313, 1.9059) (-7.9222, 2.0193) knots 0 0 0 1 2 2 2
  line L180 (-7.9222, 2.0193) -> (-7.777, 2.0193)
  line L181 (-7.777, 2.0193) -> (-7.777, 0.7577)
  line L182 (-7.777, 0.7577) -> (-7.5285, 0.7577)
  line L183 (-7.5285, 0.7577) -> (-7.5285, 0.6148)
  spline S158 degree 2 poles (-6.3861, 1.0686) (-6.3861, 0.9608) (-6.4576, 0.7781) (-6.5177, 0.7169) knots 0 0 0 1 2 2 2
  spline S159 degree 2 poles (-6.5177, 0.7169) (-6.5801, 0.6522) (-6.7366, 0.5853) (-6.8308, 0.5853) knots 0 0 0 1 2 2 2
  spline S160 degree 2 poles (-6.8308, 0.5853) (-6.925, 0.5853) (-7.0804, 0.6488) (-7.1394, 0.7123) knots 0 0 0 1 2 2 2
  spline S161 degree 2 poles (-7.1394, 0.7123) (-7.212, 0.7883) (-7.2937, 1.0436) (-7.2937, 1.2297) knots 0 0 0 1 2 2 2
  spline S162 degree 2 poles (-7.2937, 1.2297) (-7.2937, 1.4123) (-7.2188, 1.7062) (-7.1405, 1.8151) knots 0 0 0 1 2 2 2
  spline S163 degree 2 poles (-7.1405, 1.8151) (-7.0645, 1.9217) (-6.824, 2.0409) (-6.6663, 2.0409) knots 0 0 0 1 2 2 2
  spline S164 degree 2 poles (-6.6663, 2.0409) (-6.6198, 2.0409) (-6.5381, 2.0318) (-6.5075, 2.0216) knots 0 0 0 1 2 2 2
  line L184 (-6.5075, 2.0216) -> (-6.5075, 1.8412)
  line L185 (-6.5075, 1.8412) -> (-6.5154, 1.8412)
  spline S165 degree 2 poles (-6.5154, 1.8412) (-6.5415, 1.8548) (-6.6368, 1.8786) (-6.6913, 1.8786) knots 0 0 0 1 2 2 2
  spline S166 degree 2 poles (-6.6913, 1.8786) (-6.866, 1.8786) (-7.0804, 1.6426) (-7.1008, 1.4112) knots 0 0 0 1 2 2 2
  spline S167 degree 2 poles (-7.1008, 1.4112) (-7.0339, 1.4577) (-6.8932, 1.5088) (-6.8093, 1.5088) knots 0 0 0 1 2 2 2
  spline S168 degree 2 poles (-6.8093, 1.5088) (-6.7276, 1.5088) (-6.605, 1.4759) (-6.5381, 1.426) knots 0 0 0 1 2 2 2
  spline S169 degree 2 poles (-6.5381, 1.426) (-6.461, 1.3681) (-6.3861, 1.1888) (-6.3861, 1.0686) knots 0 0 0 1 2 2 2
  spline S170 degree 2 poles (-6.5767, 1.0606) (-6.5767, 1.1469) (-6.6221, 1.2637) (-6.672, 1.3046) knots 0 0 0 1 2 2 2
  spline S171 degree 2 poles (-6.672, 1.3046) (-6.7094, 1.3341) (-6.8024, 1.3533) (-6.8512, 1.3533) knots 0 0 0 1 2 2 2
  spline S172 degree 2 poles (-6.8512, 1.3533) (-6.917, 1.3533) (-7.0407, 1.3136) (-7.1008, 1.2762) knots 0 0 0 1 2 2 2
  spline S173 degree 2 poles (-7.1008, 1.2762) (-7.102, 1.2558) (-7.1042, 1.2172) (-7.1042, 1.1877) knots 0 0 0 1 2 2 2
  spline S174 degree 2 poles (-7.1042, 1.1877) (-7.1042, 1.0425) (-7.0475, 0.8644) (-7.0044, 0.8178) knots 0 0 0 1 2 2 2
  spline S175 degree 2 poles (-7.0044, 0.8178) (-6.9647, 0.7736) (-6.8785, 0.7384) (-6.8297, 0.7384) knots 0 0 0 1 2 2 2
  spline S176 degree 2 poles (-6.8297, 0.7384) (-6.7162, 0.7384) (-6.5767, 0.8995) (-6.5767, 1.0606) knots 0 0 0 1 2 2 2
  line L186 (-5.4274, 0.6148) -> (-6.1104, 0.6148)
  line L187 (-6.1104, 0.6148) -> (-6.1104, 0.7577)
  line L188 (-6.1104, 0.7577) -> (-5.8563, 0.7577)
  line L189 (-5.8563, 0.7577) -> (-5.8563, 1.696)
  line L190 (-5.8563, 1.696) -> (-6.1104, 1.696)
  line L191 (-6.1104, 1.696) -> (-6.1104, 1.8242)
  spline S177 degree 2 poles (-6.1104, 1.8242) (-5.9663, 1.8242) (-5.8302, 1.9059) (-5.8211, 2.0193) knots 0 0 0 1 2 2 2
  line L192 (-5.8211, 2.0193) -> (-5.6759, 2.0193)
  line L193 (-5.6759, 2.0193) -> (-5.6759, 0.7577)
  line L194 (-5.6759, 0.7577) -> (-5.4274, 0.7577)
  line L195 (-5.4274, 0.7577) -> (-5.4274, 0.6148)
  line L196 (-4.3768, 0.6148) -> (-5.0598, 0.6148)
  line L197 (-5.0598, 0.6148) -> (-5.0598, 0.7577)
  line L198 (-5.0598, 0.7577) -> (-4.8057, 0.7577)
  line L199 (-4.8057, 0.7577) -> (-4.8057, 1.696)
  line L200 (-4.8057, 1.696) -> (-5.0598, 1.696)
  line L201 (-5.0598, 1.696) -> (-5.0598, 1.8242)
  spline S178 degree 2 poles (-5.0598, 1.8242) (-4.9157, 1.8242) (-4.7796, 1.9059) (-4.7705, 2.0193) knots 0 0 0 1 2 2 2
  line L202 (-4.7705, 2.0193) -> (-4.6253, 2.0193)
  line L203 (-4.6253, 2.0193) -> (-4.6253, 0.7577)
  line L204 (-4.6253, 0.7577) -> (-4.3768, 0.7577)
  line L205 (-4.3768, 0.7577) -> (-4.3768, 0.6148)
  line L206 (-3.3263, 0.6148) -> (-4.0093, 0.6148)
  line L207 (-4.0093, 0.6148) -> (-4.0093, 0.7577)
  line L208 (-4.0093, 0.7577) -> (-3.7551, 0.7577)
  line L209 (-3.7551, 0.7577) -> (-3.7551, 1.696)
  line L210 (-3.7551, 1.696) -> (-4.0093, 1.696)
  line L211 (-4.0093, 1.696) -> (-4.0093, 1.8242)
  spline S179 degree 2 poles (-4.0093, 1.8242) (-3.8652, 1.8242) (-3.729, 1.9059) (-3.7199, 2.0193) knots 0 0 0 1 2 2 2
  line L212 (-3.7199, 2.0193) -> (-3.5747, 2.0193)
  line L213 (-3.5747, 2.0193) -> (-3.5747, 0.7577)
  line L214 (-3.5747, 0.7577) -> (-3.3263, 0.7577)
  line L215 (-3.3263, 0.7577) -> (-3.3263, 0.6148)
  spline S180 degree 2 poles (-2.2201, 1.0595) (-2.2201, 0.9585) (-2.2848, 0.7861) (-2.3438, 0.7225) knots 0 0 0 1 2 2 2
  spline S181 degree 2 poles (-2.3438, 0.7225) (-2.4028, 0.659) (-2.5786, 0.5853) (-2.6875, 0.5853) knots 0 0 0 1 2 2 2
  spline S182 degree 2 poles (-2.6875, 0.5853) (-2.7874, 0.5853) (-2.9825, 0.6295) (-3.054, 0.6647) knots 0 0 0 1 2 2 2
  line L216 (-3.054, 0.6647) -> (-3.054, 0.8632)
  line L217 (-3.054, 0.8632) -> (-3.0404, 0.8632)
  spline S183 degree 2 poles (-3.0404, 0.8632) (-3.0188, 0.8473) (-2.9383, 0.8065) (-2.8895, 0.7883) knots 0 0 0 1 2 2 2
  spline S184 degree 2 poles (-2.8895, 0.7883) (-2.8339, 0.7691) (-2.742, 0.7475) (-2.6841, 0.7475) knots 0 0 0 1 2 2 2
  spline S185 degree 2 poles (-2.6841, 0.7475) (-2.6274, 0.7475) (-2.5208, 0.7883) (-2.4822, 0.8326) knots 0 0 0 1 2 2 2
  spline S186 degree 2 poles (-2.4822, 0.8326) (-2.447, 0.8746) (-2.4107, 0.9858) (-2.4107, 1.0606) knots 0 0 0 1 2 2 2
  spline S187 degree 2 poles (-2.4107, 1.0606) (-2.4107, 1.1355) (-2.4516, 1.2308) (-2.4901, 1.2626) knots 0 0 0 1 2 2 2
  spline S188 degree 2 poles (-2.4901, 1.2626) (-2.5298, 1.2978) (-2.6478, 1.3272) (-2.7193, 1.3272) knots 0 0 0 1 2 2 2
  spline S189 degree 2 poles (-2.7193, 1.3272) (-2.7964, 1.3272) (-2.9496, 1.3034) (-2.9961, 1.2932) knots 0 0 0 1 2 2 2
  line L218 (-2.9961, 1.2932) -> (-2.9961, 2.0148)
  line L219 (-2.9961, 2.0148) -> (-2.2281, 2.0148)
  line L220 (-2.2281, 2.0148) -> (-2.2281, 1.8503)
  line L221 (-2.2281, 1.8503) -> (-2.8157, 1.8503)
  line L222 (-2.8157, 1.8503) -> (-2.8157, 1.477)
  spline S190 degree 2 poles (-2.8157, 1.477) (-2.7817, 1.4815) (-2.7159, 1.4849) (-2.6887, 1.4849) knots 0 0 0 1 2 2 2
  spline S191 degree 2 poles (-2.6887, 1.4849) (-2.5809, 1.4849) (-2.4323, 1.4498) (-2.3642, 1.3976) knots 0 0 0 1 2 2 2
  spline S192 degree 2 poles (-2.3642, 1.3976) (-2.295, 1.3454) (-2.2201, 1.1866) (-2.2201, 1.0595) knots 0 0 0 1 2 2 2
  line L223 (-1.5054, 1.1423) -> (-2.0352, 1.1423)
  line L224 (-2.0352, 1.1423) -> (-2.0352, 1.3125)
  line L225 (-2.0352, 1.3125) -> (-1.5054, 1.3125)
  line L226 (-1.5054, 1.3125) -> (-1.5054, 1.1423)
  spline S193 degree 2 poles (-0.4707, 1.0595) (-0.4707, 0.9585) (-0.5353, 0.7861) (-0.5943, 0.7225) knots 0 0 0 1 2 2 2
  spline S194 degree 2 poles (-0.5943, 0.7225) (-0.6533, 0.659) (-0.8292, 0.5853) (-0.9381, 0.5853) knots 0 0 0 1 2 2 2
  spline S195 degree 2 poles (-0.9381, 0.5853) (-1.0379, 0.5853) (-1.2331, 0.6295) (-1.3046, 0.6647) knots 0 0 0 1 2 2 2
  line L227 (-1.3046, 0.6647) -> (-1.3046, 0.8632)
  line L228 (-1.3046, 0.8632) -> (-1.2909, 0.8632)
  spline S196 degree 2 poles (-1.2909, 0.8632) (-1.2694, 0.8473) (-1.1888, 0.8065) (-1.14, 0.7883) knots 0 0 0 1 2 2 2
  spline S197 degree 2 poles (-1.14, 0.7883) (-1.0845, 0.7691) (-0.9926, 0.7475) (-0.9347, 0.7475) knots 0 0 0 1 2 2 2
  spline S198 degree 2 poles (-0.9347, 0.7475) (-0.878, 0.7475) (-0.7713, 0.7883) (-0.7328, 0.8326) knots 0 0 0 1 2 2 2
  spline S199 degree 2 poles (-0.7328, 0.8326) (-0.6976, 0.8746) (-0.6613, 0.9858) (-0.6613, 1.0606) knots 0 0 0 1 2 2 2
  spline S200 degree 2 poles (-0.6613, 1.0606) (-0.6613, 1.1355) (-0.7021, 1.2308) (-0.7407, 1.2626) knots 0 0 0 1 2 2 2
  spline S201 degree 2 poles (-0.7407, 1.2626) (-0.7804, 1.2978) (-0.8984, 1.3272) (-0.9699, 1.3272) knots 0 0 0 1 2 2 2
  spline S202 degree 2 poles (-0.9699, 1.3272) (-1.047, 1.3272) (-1.2002, 1.3034) (-1.2467, 1.2932) knots 0 0 0 1 2 2 2
  line L229 (-1.2467, 1.2932) -> (-1.2467, 2.0148)
  line L230 (-1.2467, 2.0148) -> (-0.4786, 2.0148)
  line L231 (-0.4786, 2.0148) -> (-0.4786, 1.8503)
  line L232 (-0.4786, 1.8503) -> (-1.0663, 1.8503)
  line L233 (-1.0663, 1.8503) -> (-1.0663, 1.477)
  spline S203 degree 2 poles (-1.0663, 1.477) (-1.0323, 1.4815) (-0.9665, 1.4849) (-0.9392, 1.4849) knots 0 0 0 1 2 2 2
  spline S204 degree 2 poles (-0.9392, 1.4849) (-0.8315, 1.4849) (-0.6828, 1.4498) (-0.6148, 1.3976) knots 0 0 0 1 2 2 2
  spline S205 degree 2 poles (-0.6148, 1.3976) (-0.5456, 1.3454) (-0.4707, 1.1866) (-0.4707, 1.0595) knots 0 0 0 1 2 2 2
  spline S206 degree 2 poles (-0.3073, 1.5598) (-0.3073, 1.6676) (-0.237, 1.8469) (-0.1757, 1.9115) knots 0 0 0 1 2 2 2
  spline S207 degree 2 poles (-0.1757, 1.9115) (-0.1178, 1.9739) (0.0512, 2.0431) (0.1374, 2.0431) knots 0 0 0 1 2 2 2
  spline S208 degree 2 poles (0.1374, 2.0431) (0.2339, 2.0431) (0.3904, 1.9785) (0.4483, 1.9172) knots 0 0 0 1 2 2 2
  spline S209 degree 2 poles (0.4483, 1.9172) (0.5209, 1.8401) (0.6003, 1.5905) (0.6003, 1.3987) knots 0 0 0 1 2 2 2
  spline S210 degree 2 poles (0.6003, 1.3987) (0.6003, 1.2251) (0.522, 0.9143) (0.446, 0.811) knots 0 0 0 1 2 2 2
  spline S211 degree 2 poles (0.446, 0.811) (0.3655, 0.7021) (0.1386, 0.5875) (-0.0271, 0.5875) knots 0 0 0 1 2 2 2
  spline S212 degree 2 poles (-0.0271, 0.5875) (-0.0645, 0.5875) (-0.1496, 0.5955) (-0.1859, 0.6068) knots 0 0 0 1 2 2 2
  line L234 (-0.1859, 0.6068) -> (-0.1859, 0.7872)
  line L235 (-0.1859, 0.7872) -> (-0.1768, 0.7872)
  spline S213 degree 2 poles (-0.1768, 0.7872) (-0.153, 0.7736) (-0.0532, 0.7498) (-0.0021, 0.7498) knots 0 0 0 1 2 2 2
  spline S214 degree 2 poles (-0.0021, 0.7498) (0.1817, 0.7498) (0.3916, 0.9926) (0.4063, 1.2172) knots 0 0 0 1 2 2 2
  spline S215 degree 2 poles (0.4063, 1.2172) (0.3314, 1.1661) (0.1953, 1.1196) (0.1147, 1.1196) knots 0 0 0 1 2 2 2
  spline S216 degree 2 poles (0.1147, 1.1196) (0.0376, 1.1196) (-0.0906, 1.1537) (-0.1553, 1.2025) knots 0 0 0 1 2 2 2
  spline S217 degree 2 poles (-0.1553, 1.2025) (-0.2302, 1.2603) (-0.3073, 1.4362) (-0.3073, 1.5598) knots 0 0 0 1 2 2 2
  spline S218 degree 2 poles (0.4108, 1.4407) (0.4108, 1.5825) (0.3587, 1.7618) (0.3121, 1.8106) knots 0 0 0 1 2 2 2
  spline S219 degree 2 poles (0.3121, 1.8106) (0.2713, 1.8559) (0.1862, 1.89) (0.1363, 1.89) knots 0 0 0 1 2 2 2
  spline S220 degree 2 poles (0.1363, 1.89) (0.0206, 1.89) (-0.1167, 1.7243) (-0.1167, 1.5678) knots 0 0 0 1 2 2 2
  spline S221 degree 2 poles (-0.1167, 1.5678) (-0.1167, 1.4793) (-0.0713, 1.3647) (-0.0214, 1.3238) knots 0 0 0 1 2 2 2
  spline S222 degree 2 poles (-0.0214, 1.3238) (0.0149, 1.2943) (0.1045, 1.2751) (0.1567, 1.2751) knots 0 0 0 1 2 2 2
  spline S223 degree 2 poles (0.1567, 1.2751) (0.2168, 1.2751) (0.3553, 1.317) (0.4074, 1.3522) knots 0 0 0 1 2 2 2
  spline S224 degree 2 poles (0.4074, 1.3522) (0.4086, 1.3658) (0.4108, 1.4123) (0.4108, 1.4407) knots 0 0 0 1 2 2 2
  spline S225 degree 2 poles (-12.7122, -1.7153) (-12.8483, -1.7153) (-13.0786, -1.6234) (-13.1626, -1.5315) knots 0 0 0 1 2 2 2
  spline S226 degree 2 poles (-13.1626, -1.5315) (-13.2465, -1.4407) (-13.3384, -1.1684) (-13.3384, -0.9914) knots 0 0 0 1 2 2 2
  spline S227 degree 2 poles (-13.3384, -0.9914) (-13.3384, -0.8156) (-13.2488, -0.5546) (-13.1637, -0.4582) knots 0 0 0 1 2 2 2
  spline S228 degree 2 poles (-13.1637, -0.4582) (-13.0798, -0.364) (-12.8506, -0.2653) (-12.7088, -0.2653) knots 0 0 0 1 2 2 2
  spline S229 degree 2 poles (-12.7088, -0.2653) (-12.6384, -0.2653) (-12.5148, -0.2858) (-12.4626, -0.3016) knots 0 0 0 1 2 2 2
  spline S230 degree 2 poles (-12.4626, -0.3016) (-12.4172, -0.3164) (-12.323, -0.3584) (-12.2765, -0.3833) knots 0 0 0 1 2 2 2
  line L236 (-12.2765, -0.3833) -> (-12.2765, -0.608)
  line L237 (-12.2765, -0.608) -> (-12.2913, -0.608)
  spline S231 degree 2 poles (-12.2913, -0.608) (-12.3162, -0.5853) (-12.3934, -0.5217) (-12.449, -0.4911) knots 0 0 0 1 2 2 2
  spline S232 degree 2 poles (-12.449, -0.4911) (-12.5023, -0.4616) (-12.6282, -0.4242) (-12.7099, -0.4242) knots 0 0 0 1 2 2 2
  spline S233 degree 2 poles (-12.7099, -0.4242) (-12.7995, -0.4242) (-12.9595, -0.4979) (-13.0196, -0.5683) knots 0 0 0 1 2 2 2
  spline S234 degree 2 poles (-13.0196, -0.5683) (-13.0786, -0.6397) (-13.1444, -0.8564) (-13.1444, -0.9914) knots 0 0 0 1 2 2 2
  spline S235 degree 2 poles (-13.1444, -0.9914) (-13.1444, -1.1355) (-13.0752, -1.3431) (-13.0151, -1.4146) knots 0 0 0 1 2 2 2
  spline S236 degree 2 poles (-13.0151, -1.4146) (-12.9561, -1.4838) (-12.7984, -1.5542) (-12.7099, -1.5542) knots 0 0 0 1 2 2 2
  spline S237 degree 2 poles (-12.7099, -1.5542) (-12.6293, -1.5542) (-12.4921, -1.5144) (-12.4387, -1.4849) knots 0 0 0 1 2 2 2
  spline S238 degree 2 poles (-12.4387, -1.4849) (-12.3877, -1.4554) (-12.3117, -1.3942) (-12.2901, -1.3726) knots 0 0 0 1 2 2 2
  line L238 (-12.2901, -1.3726) -> (-12.2765, -1.3726)
  line L239 (-12.2765, -1.3726) -> (-12.2765, -1.595)
  spline S239 degree 2 poles (-12.2765, -1.595) (-12.323, -1.6166) (-12.4047, -1.6563) (-12.4626, -1.6744) knots 0 0 0 1 2 2 2
  spline S240 degree 2 poles (-12.4626, -1.6744) (-12.5238, -1.6948) (-12.6282, -1.7153) (-12.7122, -1.7153) knots 0 0 0 1 2 2 2
  spline S241 degree 2 poles (-11.6605, -1.7141) (-11.9123, -1.7141) (-12.1892, -1.4316) (-12.1892, -1.1707) knots 0 0 0 1 2 2 2
  spline S242 degree 2 poles (-12.1892, -1.1707) (-12.1892, -0.9143) (-11.9203, -0.6102) (-11.7036, -0.6102) knots 0 0 0 1 2 2 2
  spline S243 degree 2 poles (-11.7036, -0.6102) (-11.606, -0.6102) (-11.4551, -0.667) (-11.3995, -0.7271) knots 0 0 0 1 2 2 2
  spline S244 degree 2 poles (-11.3995, -0.7271) (-11.3428, -0.7872) (-11.2827, -0.9608) (-11.2827, -1.0867) knots 0 0 0 1 2 2 2
  line L240 (-11.2827, -1.0867) -> (-11.2827, -1.1832)
  line L241 (-11.2827, -1.1832) -> (-12.0099, -1.1832)
  spline S245 degree 2 poles (-12.0099, -1.1832) (-12.0099, -1.3658) (-11.8261, -1.5598) (-11.6627, -1.5598) knots 0 0 0 1 2 2 2
  spline S246 degree 2 poles (-11.6627, -1.5598) (-11.6049, -1.5598) (-11.4926, -1.5337) (-11.4472, -1.5133) knots 0 0 0 1 2 2 2
  spline S247 degree 2 poles (-11.4472, -1.5133) (-11.3995, -1.4906) (-11.3337, -1.4509) (-11.3122, -1.4328) knots 0 0 0 1 2 2 2
  line L242 (-11.3122, -1.4328) -> (-11.302, -1.4328)
  line L243 (-11.302, -1.4328) -> (-11.302, -1.6256)
  spline S248 degree 2 poles (-11.302, -1.6256) (-11.3326, -1.6381) (-11.4256, -1.6744) (-11.4619, -1.6846) knots 0 0 0 1 2 2 2
  spline S249 degree 2 poles (-11.4619, -1.6846) (-11.513, -1.6994) (-11.5969, -1.7141) (-11.6605, -1.7141) knots 0 0 0 1 2 2 2
  spline S250 degree 2 poles (-11.4551, -1.0482) (-11.4574, -0.9767) (-11.4869, -0.8723) (-11.5152, -0.8371) knots 0 0 0 1 2 2 2
  spline S251 degree 2 poles (-11.5152, -0.8371) (-11.5459, -0.7974) (-11.6423, -0.7554) (-11.7138, -0.7554) knots 0 0 0 1 2 2 2
  spline S252 degree 2 poles (-11.7138, -0.7554) (-11.7841, -0.7554) (-11.8828, -0.7974) (-11.9237, -0.8383) knots 0 0 0 1 2 2 2
  spline S253 degree 2 poles (-11.9237, -0.8383) (-11.9634, -0.8802) (-12.0042, -0.9812) (-12.0099, -1.0482) knots 0 0 0 1 2 2 2
  line L244 (-12.0099, -1.0482) -> (-11.4551, -1.0482)
  line L245 (-10.2786, -1.6903) -> (-10.4556, -1.6903)
  line L246 (-10.4556, -1.6903) -> (-10.4556, -1.0913)
  spline S254 degree 2 poles (-10.4556, -1.0913) (-10.4556, -1.0187) (-10.4692, -0.8939) (-10.4896, -0.8564) knots 0 0 0 1 2 2 2
  spline S255 degree 2 poles (-10.4896, -0.8564) (-10.5112, -0.8167) (-10.5883, -0.7781) (-10.6541, -0.7781) knots 0 0 0 1 2 2 2
  spline S256 degree 2 poles (-10.6541, -0.7781) (-10.7199, -0.7781) (-10.8595, -0.8485) (-10.9264, -0.9052) knots 0 0 0 1 2 2 2
  line L247 (-10.9264, -0.9052) -> (-10.9264, -1.6903)
  line L248 (-10.9264, -1.6903) -> (-11.1034, -1.6903)
  line L249 (-11.1034, -1.6903) -> (-11.1034, -0.6397)
  line L250 (-11.1034, -0.6397) -> (-10.9264, -0.6397)
  line L251 (-10.9264, -0.6397) -> (-10.9264, -0.7566)
  spline S257 degree 2 poles (-10.9264, -0.7566) (-10.847, -0.6851) (-10.6939, -0.6102) (-10.6076, -0.6102) knots 0 0 0 1 2 2 2
  spline S258 degree 2 poles (-10.6076, -0.6102) (-10.4533, -0.6102) (-10.2786, -0.8144) (-10.2786, -1.0084) knots 0 0 0 1 2 2 2
  line L252 (-10.2786, -1.0084) -> (-10.2786, -1.6903)
  spline S259 degree 2 poles (-9.7125, -1.7107) (-9.8566, -1.7107) (-10.0188, -1.5462) (-10.0188, -1.3681) knots 0 0 0 1 2 2 2
  line L253 (-10.0188, -1.3681) -> (-10.0188, -0.7861)
  line L254 (-10.0188, -0.7861) -> (-10.1379, -0.7861)
  line L255 (-10.1379, -0.7861) -> (-10.1379, -0.6397)
  line L256 (-10.1379, -0.6397) -> (-10.0188, -0.6397)
  line L257 (-10.0188, -0.6397) -> (-10.0188, -0.3379)
  line L258 (-10.0188, -0.3379) -> (-9.8418, -0.3379)
  line L259 (-9.8418, -0.3379) -> (-9.8418, -0.6397)
  line L260 (-9.8418, -0.6397) -> (-9.5162, -0.6397)
  line L261 (-9.5162, -0.6397) -> (-9.5162, -0.7861)
  line L262 (-9.5162, -0.7861) -> (-9.8418, -0.7861)
  line L263 (-9.8418, -0.7861) -> (-9.8418, -1.2864)
  spline S260 degree 2 poles (-9.8418, -1.2864) (-9.8418, -1.3658) (-9.8362, -1.4532) (-9.8169, -1.4906) knots 0 0 0 1 2 2 2
  spline S261 degree 2 poles (-9.8169, -1.4906) (-9.801, -1.5235) (-9.7295, -1.5564) (-9.6682, -1.5564) knots 0 0 0 1 2 2 2
  spline S262 degree 2 poles (-9.6682, -1.5564) (-9.6251, -1.5564) (-9.5446, -1.5303) (-9.5264, -1.5224) knots 0 0 0 1 2 2 2
  line L264 (-9.5264, -1.5224) -> (-9.5162, -1.5224)
  line L265 (-9.5162, -1.5224) -> (-9.5162, -1.6812)
  spline S263 degree 2 poles (-9.5162, -1.6812) (-9.5661, -1.6948) (-9.6682, -1.7107) (-9.7125, -1.7107) knots 0 0 0 1 2 2 2
  spline S264 degree 2 poles (-8.9297, -1.7141) (-9.1815, -1.7141) (-9.4584, -1.4316) (-9.4584, -1.1707) knots 0 0 0 1 2 2 2
  spline S265 degree 2 poles (-9.4584, -1.1707) (-9.4584, -0.9143) (-9.1895, -0.6102) (-8.9728, -0.6102) knots 0 0 0 1 2 2 2
  spline S266 degree 2 poles (-8.9728, -0.6102) (-8.8752, -0.6102) (-8.7243, -0.667) (-8.6687, -0.7271) knots 0 0 0 1 2 2 2
  spline S267 degree 2 poles (-8.6687, -0.7271) (-8.612, -0.7872) (-8.5519, -0.9608) (-8.5519, -1.0867) knots 0 0 0 1 2 2 2
  line L266 (-8.5519, -1.0867) -> (-8.5519, -1.1832)
  line L267 (-8.5519, -1.1832) -> (-9.2791, -1.1832)
  spline S268 degree 2 poles (-9.2791, -1.1832) (-9.2791, -1.3658) (-9.0953, -1.5598) (-8.9319, -1.5598) knots 0 0 0 1 2 2 2
  spline S269 degree 2 poles (-8.9319, -1.5598) (-8.8741, -1.5598) (-8.7618, -1.5337) (-8.7164, -1.5133) knots 0 0 0 1 2 2 2
  spline S270 degree 2 poles (-8.7164, -1.5133) (-8.6687, -1.4906) (-8.6029, -1.4509) (-8.5814, -1.4328) knots 0 0 0 1 2 2 2
  line L268 (-8.5814, -1.4328) -> (-8.5712, -1.4328)
  line L269 (-8.5712, -1.4328) -> (-8.5712, -1.6256)
  spline S271 degree 2 poles (-8.5712, -1.6256) (-8.6018, -1.6381) (-8.6948, -1.6744) (-8.7311, -1.6846) knots 0 0 0 1 2 2 2
  spline S272 degree 2 poles (-8.7311, -1.6846) (-8.7822, -1.6994) (-8.8661, -1.7141) (-8.9297, -1.7141) knots 0 0 0 1 2 2 2
  spline S273 degree 2 poles (-8.7243, -1.0482) (-8.7266, -0.9767) (-8.7561, -0.8723) (-8.7845, -0.8371) knots 0 0 0 1 2 2 2
  spline S274 degree 2 poles (-8.7845, -0.8371) (-8.8151, -0.7974) (-8.9115, -0.7554) (-8.983, -0.7554) knots 0 0 0 1 2 2 2
  spline S275 degree 2 poles (-8.983, -0.7554) (-9.0533, -0.7554) (-9.152, -0.7974) (-9.1929, -0.8383) knots 0 0 0 1 2 2 2
  spline S276 degree 2 poles (-9.1929, -0.8383) (-9.2326, -0.8802) (-9.2734, -0.9812) (-9.2791, -1.0482) knots 0 0 0 1 2 2 2
  line L270 (-9.2791, -1.0482) -> (-8.7243, -1.0482)
  line L271 (-7.8156, -0.8292) -> (-7.8246, -0.8292)
  spline S277 degree 2 poles (-7.8246, -0.8292) (-7.8451, -0.8235) (-7.8893, -0.8213) (-7.9199, -0.8213) knots 0 0 0 1 2 2 2
  spline S278 degree 2 poles (-7.9199, -0.8213) (-7.9914, -0.8213) (-8.1321, -0.8836) (-8.1956, -0.9449) knots 0 0 0 1 2 2 2
  line L272 (-8.1956, -0.9449) -> (-8.1956, -1.6903)
  line L273 (-8.1956, -1.6903) -> (-8.3726, -1.6903)
  line L274 (-8.3726, -1.6903) -> (-8.3726, -0.6397)
  line L275 (-8.3726, -0.6397) -> (-8.1956, -0.6397)
  line L276 (-8.1956, -0.6397) -> (-8.1956, -0.7963)
  spline S279 degree 2 poles (-8.1956, -0.7963) (-8.0992, -0.7101) (-7.9551, -0.6397) (-7.887, -0.6397) knots 0 0 0 1 2 2 2
  spline S280 degree 2 poles (-7.887, -0.6397) (-7.8598, -0.6397) (-7.8326, -0.642) (-7.8156, -0.6454) knots 0 0 0 1 2 2 2
  line L277 (-7.8156, -0.6454) -> (-7.8156, -0.8292)
  line L278 (-5.4943, -0.2903) -> (-5.846, -1.6903)
  line L279 (-5.846, -1.6903) -> (-6.0548, -1.6903)